Autodesk Inventor part; units mm, degrees
(part 2 of 2)
sketch "Sketch11" plane through (0, 0, 0) normal (0, -1, 0) x (1, 0, 0)
  line L0 (38.5, 57.5) -> (38.5, -57.5) construction
  line L1 (-38.5, 57.5) -> (38.5, 57.5) construction
  line L2 (-38.5, 57.5) -> (-38.5, -57.5) construction
  line L3 (-38.5, -57.5) -> (38.5, -57.5) construction
  line L4 (-32.0325, -46.9289) -> (-28.4969, -50.4645)
  line L5 (-28.4969, -50.4645) -> (-32.0325, -54)
  line L6 (-32.0325, -54) -> (-35.568, -50.4645)
  line L7 (-35.568, -50.4645) -> (-32.0325, -46.9289)
  line L8 (-38.5, -54) -> (-32.0325, -54) construction
  line L9 (31.4645, 54) -> (35, 54) construction
  line L10 (-38.5, -54) -> (35, -54) construction
  line L11 (35, 54) -> (-38.5, 54)
  line L12 (-38.5, 54) -> (-38.5, -54) construction
  line L13 (-22.9615, -46.9289) -> (-19.4259, -50.4645)
  line L14 (-26.497, -50.4645) -> (-22.9615, -46.9289)
  line L15 (-19.4259, -50.4645) -> (-22.9615, -54)
  line L16 (-22.9615, -54) -> (-26.497, -50.4645)
  line L17 (-13.8905, -46.9289) -> (-10.3549, -50.4645)
  line L18 (-17.426, -50.4645) -> (-13.8905, -46.9289)
  line L19 (-10.3549, -50.4645) -> (-13.8905, -54)
  line L20 (-13.8905, -54) -> (-17.426, -50.4645)
  line L21 (-4.8195, -46.9289) -> (-1.2839, -50.4645)
  line L22 (-8.355, -50.4645) -> (-4.8195, -46.9289)
  line L23 (-1.2839, -50.4645) -> (-4.8195, -54)
  line L24 (-4.8195, -54) -> (-8.355, -50.4645)
  line L25 (4.2515, -46.9289) -> (7.7871, -50.4645)
  line L26 (0.716, -50.4645) -> (4.2515, -46.9289)
  line L27 (7.7871, -50.4645) -> (4.2515, -54)
  line L28 (4.2515, -54) -> (0.716, -50.4645)
  line L29 (13.3225, -46.9289) -> (16.8581, -50.4645)
  line L30 (9.787, -50.4645) -> (13.3225, -46.9289)
  line L31 (16.8581, -50.4645) -> (13.3225, -54)
  line L32 (13.3225, -54) -> (9.787, -50.4645)
  line L33 (22.3935, -46.9289) -> (25.9291, -50.4645)
  line L34 (18.858, -50.4645) -> (22.3935, -46.9289)
  line L35 (25.9291, -50.4645) -> (22.3935, -54)
  line L36 (22.3935, -54) -> (18.858, -50.4645)
  line L37 (31.4645, -46.9289) -> (35.0001, -50.4645)
  line L38 (27.929, -50.4645) -> (31.4645, -46.9289)
  line L39 (35.0001, -50.4645) -> (31.4645, -54)
  line L40 (31.4645, -54) -> (27.929, -50.4645)
  line L41 (-32.0325, -37.9489) -> (-28.4969, -41.4845)
  line L42 (-35.568, -41.4845) -> (-32.0325, -37.9489)
  line L43 (-28.4969, -41.4845) -> (-32.0325, -45.02)
  line L44 (-32.0325, -45.02) -> (-35.568, -41.4845)
  line L45 (-22.9615, -37.9489) -> (-19.4259, -41.4845)
  line L46 (-26.497, -41.4845) -> (-22.9615, -37.9489)
  line L47 (-19.4259, -41.4845) -> (-22.9615, -45.02)
  line L48 (-22.9615, -45.02) -> (-26.497, -41.4845)
  line L49 (-13.8905, -37.9489) -> (-10.3549, -41.4845)
  line L50 (-17.426, -41.4845) -> (-13.8905, -37.9489)
  line L51 (-10.3549, -41.4845) -> (-13.8905, -45.02)
  line L52 (-13.8905, -45.02) -> (-17.426, -41.4845)
  line L53 (-4.8195, -37.9489) -> (-1.2839, -41.4845)
  line L54 (-8.355, -41.4845) -> (-4.8195, -37.9489)
  line L55 (-1.2839, -41.4845) -> (-4.8195, -45.02)
  line L56 (-4.8195, -45.02) -> (-8.355, -41.4845)
  line L57 (4.2515, -37.9489) -> (7.7871, -41.4845)
  line L58 (0.716, -41.4845) -> (4.2515, -37.9489)
  line L59 (7.7871, -41.4845) -> (4.2515, -45.02)
  line L60 (4.2515, -45.02) -> (0.716, -41.4845)
  line L61 (13.3225, -37.9489) -> (16.8581, -41.4845)
  line L62 (9.787, -41.4845) -> (13.3225, -37.9489)
  line L63 (16.8581, -41.4845) -> (13.3225, -45.02)
  line L64 (13.3225, -45.02) -> (9.787, -41.4845)
  line L65 (22.3935, -37.9489) -> (25.9291, -41.4845)
  line L66 (18.858, -41.4845) -> (22.3935, -37.9489)
  line L67 (25.9291, -41.4845) -> (22.3935, -45.02)
  line L68 (22.3935, -45.02) -> (18.858, -41.4845)
  line L69 (31.4645, -37.9489) -> (35.0001, -41.4845)
  line L70 (27.929, -41.4845) -> (31.4645, -37.9489)
  line L71 (35.0001, -41.4845) -> (31.4645, -45.02)
  line L72 (31.4645, -45.02) -> (27.929, -41.4845)
  line L73 (-32.0325, -28.9689) -> (-28.4969, -32.5045)
  line L74 (-35.568, -32.5045) -> (-32.0325, -28.9689)
  line L75 (-28.4969, -32.5045) -> (-32.0325, -36.04)
  line L76 (-32.0325, -36.04) -> (-35.568, -32.5045)
  line L77 (-22.9615, -28.9689) -> (-19.4259, -32.5045)
  line L78 (-26.497, -32.5045) -> (-22.9615, -28.9689)
  line L79 (-19.4259, -32.5045) -> (-22.9615, -36.04)
  line L80 (-22.9615, -36.04) -> (-26.497, -32.5045)
  line L81 (-13.8905, -28.9689) -> (-10.3549, -32.5045)
  line L82 (-17.426, -32.5045) -> (-13.8905, -28.9689)
  line L83 (-10.3549, -32.5045) -> (-13.8905, -36.04)
  line L84 (-13.8905, -36.04) -> (-17.426, -32.5045)
  line L85 (-4.8195, -28.9689) -> (-1.2839, -32.5045)
  line L86 (-8.355, -32.5045) -> (-4.8195, -28.9689)
  line L87 (-1.2839, -32.5045) -> (-4.8195, -36.04)
  line L88 (-4.8195, -36.04) -> (-8.355, -32.5045)
  line L89 (4.2515, -28.9689) -> (7.7871, -32.5045)
  line L90 (0.716, -32.5045) -> (4.2515, -28.9689)
  line L91 (7.7871, -32.5045) -> (4.2515, -36.04)
  line L92 (4.2515, -36.04) -> (0.716, -32.5045)
  line L93 (13.3225, -28.9689) -> (16.8581, -32.5045)
  line L94 (9.787, -32.5045) -> (13.3225, -28.9689)
  line L95 (16.8581, -32.5045) -> (13.3225, -36.04)
  line L96 (13.3225, -36.04) -> (9.787, -32.5045)
  line L97 (22.3935, -28.9689) -> (25.9291, -32.5045)
  line L98 (18.858, -32.5045) -> (22.3935, -28.9689)
  line L99 (25.9291, -32.5045) -> (22.3935, -36.04)
  line L100 (22.3935, -36.04) -> (18.858, -32.5045)
  line L101 (31.4645, -28.9689) -> (35.0001, -32.5045)
  line L102 (27.929, -32.5045) -> (31.4645, -28.9689)
  line L103 (35.0001, -32.5045) -> (31.4645, -36.04)
  line L104 (31.4645, -36.04) -> (27.929, -32.5045)
  line L105 (-32.0325, -19.9889) -> (-28.4969, -23.5245)
  line L106 (-35.568, -23.5245) -> (-32.0325, -19.9889)
  line L107 (-28.4969, -23.5245) -> (-32.0325, -27.06)
  line L108 (-32.0325, -27.06) -> (-35.568, -23.5245)
  line L109 (-22.9615, -19.9889) -> (-19.4259, -23.5245)
  line L110 (-26.497, -23.5245) -> (-22.9615, -19.9889)
  line L111 (-19.4259, -23.5245) -> (-22.9615, -27.06)
  line L112 (-22.9615, -27.06) -> (-26.497, -23.5245)
  line L113 (-13.8905, -19.9889) -> (-10.3549, -23.5245)
  line L114 (-17.426, -23.5245) -> (-13.8905, -19.9889)
  line L115 (-10.3549, -23.5245) -> (-13.8905, -27.06)
  line L116 (-13.8905, -27.06) -> (-17.426, -23.5245)
  line L117 (-4.8195, -19.9889) -> (-1.2839, -23.5245)
  line L118 (-8.355, -23.5245) -> (-4.8195, -19.9889)
  line L119 (-1.2839, -23.5245) -> (-4.8195, -27.06)
  line L120 (-4.8195, -27.06) -> (-8.355, -23.5245)
  line L121 (4.2515, -19.9889) -> (7.7871, -23.5245)
  line L122 (0.716, -23.5245) -> (4.2515, -19.9889)
  line L123 (7.7871, -23.5245) -> (4.2515, -27.06)
  line L124 (4.2515, -27.06) -> (0.716, -23.5245)
  line L125 (13.3225, -19.9889) -> (16.8581, -23.5245)
  line L126 (9.787, -23.5245) -> (13.3225, -19.9889)
  line L127 (16.8581, -23.5245) -> (13.3225, -27.06)
  line L128 (13.3225, -27.06) -> (9.787, -23.5245)
  line L129 (22.3935, -19.9889) -> (25.9291, -23.5245)
  line L130 (18.858, -23.5245) -> (22.3935, -19.9889)
  line L131 (25.9291, -23.5245) -> (22.3935, -27.06)
  line L132 (22.3935, -27.06) -> (18.858, -23.5245)
  line L133 (31.4645, -19.9889) -> (35.0001, -23.5245)
  line L134 (27.929, -23.5245) -> (31.4645, -19.9889)
  line L135 (35.0001, -23.5245) -> (31.4645, -27.06)
  line L136 (31.4645, -27.06) -> (27.929, -23.5245)
  line L137 (-32.0325, -11.0089) -> (-28.4969, -14.5445)
  line L138 (-35.568, -14.5445) -> (-32.0325, -11.0089)
  line L139 (-28.4969, -14.5445) -> (-32.0325, -18.08)
  line L140 (-32.0325, -18.08) -> (-35.568, -14.5445)
  line L141 (-22.9615, -11.0089) -> (-19.4259, -14.5445)
  line L142 (-26.497, -14.5445) -> (-22.9615, -11.0089)
  line L143 (-19.4259, -14.5445) -> (-22.9615, -18.08)
  line L144 (-22.9615, -18.08) -> (-26.497, -14.5445)
  line L145 (-13.8905, -11.0089) -> (-10.3549, -14.5445)
  line L146 (-17.426, -14.5445) -> (-13.8905, -11.0089)
  line L147 (-10.3549, -14.5445) -> (-13.8905, -18.08)
  line L148 (-13.8905, -18.08) -> (-17.426, -14.5445)
  line L149 (-4.8195, -11.0089) -> (-1.2839, -14.5445)
  line L150 (-8.355, -14.5445) -> (-4.8195, -11.0089)
  line L151 (-1.2839, -14.5445) -> (-4.8195, -18.08)
  line L152 (-4.8195, -18.08) -> (-8.355, -14.5445)
  line L153 (4.2515, -11.0089) -> (7.7871, -14.5445)
  line L154 (0.716, -14.5445) -> (4.2515, -11.0089)
  line L155 (7.7871, -14.5445) -> (4.2515, -18.08)
  line L156 (4.2515, -18.08) -> (0.716, -14.5445)
  line L157 (13.3225, -11.0089) -> (16.8581, -14.5445)
  line L158 (9.787, -14.5445) -> (13.3225, -11.0089)
  line L159 (16.8581, -14.5445) -> (13.3225, -18.08)
  line L160 (13.3225, -18.08) -> (9.787, -14.5445)
  line L161 (22.3935, -11.0089) -> (25.9291, -14.5445)
  line L162 (18.858, -14.5445) -> (22.3935, -11.0089)
  line L163 (25.9291, -14.5445) -> (22.3935, -18.08)
  line L164 (22.3935, -18.08) -> (18.858, -14.5445)
  line L165 (31.4645, -11.0089) -> (35.0001, -14.5445)
  line L166 (27.929, -14.5445) -> (31.4645, -11.0089)
  line L167 (35.0001, -14.5445) -> (31.4645, -18.08)
  line L168 (31.4645, -18.08) -> (27.929, -14.5445)
  line L169 (-38.5, -57.5) -> (-38.5, 57.5) construction
  line L170 (-38.5, 0) -> (38.5, 0) construction
  line L171 (38.5, 57.5) -> (38.5, -57.5) construction
  line L172 (-31.0325, -45.9745) -> (-27.497, -49.51)
  line L173 (-27.497, -49.51) -> (-23.9614, -45.9745)
  line L174 (-23.9614, -45.9745) -> (-27.497, -42.4389)
  line L175 (-27.497, -42.4389) -> (-31.0325, -45.9745)
  line L176 (-18.426, -49.51) -> (-14.8904, -45.9745)
  line L177 (-14.8904, -45.9745) -> (-18.426, -42.4389)
  line L178 (-21.9615, -45.9745) -> (-18.426, -49.51)
  line L179 (-18.426, -42.4389) -> (-21.9615, -45.9745)
  line L180 (-9.355, -49.51) -> (-5.8194, -45.9745)
  line L181 (-5.8194, -45.9745) -> (-9.355, -42.4389)
  line L182 (-12.8905, -45.9745) -> (-9.355, -49.51)
  line L183 (-9.355, -42.4389) -> (-12.8905, -45.9745)
  line L184 (-0.284, -49.51) -> (3.2516, -45.9745)
  line L185 (3.2516, -45.9745) -> (-0.284, -42.4389)
  line L186 (-3.8195, -45.9745) -> (-0.284, -49.51)
  line L187 (-0.284, -42.4389) -> (-3.8195, -45.9745)
  line L188 (8.787, -49.51) -> (12.3226, -45.9745)
  line L189 (12.3226, -45.9745) -> (8.787, -42.4389)
  line L190 (5.2515, -45.9745) -> (8.787, -49.51)
  line L191 (8.787, -42.4389) -> (5.2515, -45.9745)
  line L192 (17.858, -49.51) -> (21.3936, -45.9745)
  line L193 (21.3936, -45.9745) -> (17.858, -42.4389)
  line L194 (14.3225, -45.9745) -> (17.858, -49.51)
  line L195 (17.858, -42.4389) -> (14.3225, -45.9745)
  line L196 (26.929, -49.51) -> (30.4646, -45.9745)
  line L197 (30.4646, -45.9745) -> (26.929, -42.4389)
  line L198 (23.3935, -45.9745) -> (26.929, -49.51)
  line L199 (26.929, -42.4389) -> (23.3935, -45.9745)
  line L200 (-27.497, -40.53) -> (-23.9614, -36.9945)
  line L201 (-23.9614, -36.9945) -> (-27.497, -33.4589)
  line L202 (-31.0325, -36.9945) -> (-27.497, -40.53)
  line L203 (-27.497, -33.4589) -> (-31.0325, -36.9945)
  line L204 (-18.426, -40.53) -> (-14.8904, -36.9945)
  line L205 (-14.8904, -36.9945) -> (-18.426, -33.4589)
  line L206 (-21.9615, -36.9945) -> (-18.426, -40.53)
  line L207 (-18.426, -33.4589) -> (-21.9615, -36.9945)
  line L208 (-9.355, -40.53) -> (-5.8194, -36.9945)
  line L209 (-5.8194, -36.9945) -> (-9.355, -33.4589)
  line L210 (-12.8905, -36.9945) -> (-9.355, -40.53)
  line L211 (-9.355, -33.4589) -> (-12.8905, -36.9945)
  line L212 (-0.284, -40.53) -> (3.2516, -36.9945)
  line L213 (3.2516, -36.9945) -> (-0.284, -33.4589)
  line L214 (-3.8195, -36.9945) -> (-0.284, -40.53)
  line L215 (-0.284, -33.4589) -> (-3.8195, -36.9945)
  line L216 (8.787, -40.53) -> (12.3226, -36.9945)
  line L217 (12.3226, -36.9945) -> (8.787, -33.4589)
  line L218 (5.2515, -36.9945) -> (8.787, -40.53)
  line L219 (8.787, -33.4589) -> (5.2515, -36.9945)
  line L220 (17.858, -40.53) -> (21.3936, -36.9945)
  line L221 (21.3936, -36.9945) -> (17.858, -33.4589)
  line L222 (14.3225, -36.9945) -> (17.858, -40.53)
  line L223 (17.858, -33.4589) -> (14.3225, -36.9945)
  line L224 (26.929, -40.53) -> (30.4646, -36.9945)
  line L225 (30.4646, -36.9945) -> (26.929, -33.4589)
  line L226 (23.3935, -36.9945) -> (26.929, -40.53)
  line L227 (26.929, -33.4589) -> (23.3935, -36.9945)
  line L228 (-27.497, -31.55) -> (-23.9614, -28.0145)
  line L229 (-23.9614, -28.0145) -> (-27.497, -24.4789)
  line L230 (-31.0325, -28.0145) -> (-27.497, -31.55)
  line L231 (-27.497, -24.4789) -> (-31.0325, -28.0145)
  line L232 (-18.426, -31.55) -> (-14.8904, -28.0145)
  line L233 (-14.8904, -28.0145) -> (-18.426, -24.4789)
  line L234 (-21.9615, -28.0145) -> (-18.426, -31.55)
  line L235 (-18.426, -24.4789) -> (-21.9615, -28.0145)
  line L236 (-9.355, -31.55) -> (-5.8194, -28.0145)
  line L237 (-5.8194, -28.0145) -> (-9.355, -24.4789)
  line L238 (-12.8905, -28.0145) -> (-9.355, -31.55)
  line L239 (-9.355, -24.4789) -> (-12.8905, -28.0145)
  line L240 (-0.284, -31.55) -> (3.2516, -28.0145)
  line L241 (3.2516, -28.0145) -> (-0.284, -24.4789)
  line L242 (-3.8195, -28.0145) -> (-0.284, -31.55)
  line L243 (-0.284, -24.4789) -> (-3.8195, -28.0145)
  line L244 (8.787, -31.55) -> (12.3226, -28.0145)
  line L245 (12.3226, -28.0145) -> (8.787, -24.4789)
  line L246 (5.2515, -28.0145) -> (8.787, -31.55)
  line L247 (8.787, -24.4789) -> (5.2515, -28.0145)
  line L248 (17.858, -31.55) -> (21.3936, -28.0145)
  line L249 (21.3936, -28.0145) -> (17.858, -24.4789)
  line L250 (14.3225, -28.0145) -> (17.858, -31.55)
  line L251 (17.858, -24.4789) -> (14.3225, -28.0145)
  line L252 (26.929, -31.55) -> (30.4646, -28.0145)
  line L253 (30.4646, -28.0145) -> (26.929, -24.4789)
  line L254 (23.3935, -28.0145) -> (26.929, -31.55)
  line L255 (26.929, -24.4789) -> (23.3935, -28.0145)
  line L256 (-27.497, -22.57) -> (-23.9614, -19.0345)
  line L257 (-23.9614, -19.0345) -> (-27.497, -15.4989)
  line L258 (-31.0325, -19.0345) -> (-27.497, -22.57)
  line L259 (-27.497, -15.4989) -> (-31.0325, -19.0345)
  line L260 (-18.426, -22.57) -> (-14.8904, -19.0345)
  line L261 (-14.8904, -19.0345) -> (-18.426, -15.4989)
  line L262 (-21.9615, -19.0345) -> (-18.426, -22.57)
  line L263 (-18.426, -15.4989) -> (-21.9615, -19.0345)
  line L264 (-9.355, -22.57) -> (-5.8194, -19.0345)
  line L265 (-5.8194, -19.0345) -> (-9.355, -15.4989)
  line L266 (-12.8905, -19.0345) -> (-9.355, -22.57)
  line L267 (-9.355, -15.4989) -> (-12.8905, -19.0345)
  line L268 (-0.284, -22.57) -> (3.2516, -19.0345)
  line L269 (3.2516, -19.0345) -> (-0.284, -15.4989)
  line L270 (-3.8195, -19.0345) -> (-0.284, -22.57)
  line L271 (-0.284, -15.4989) -> (-3.8195, -19.0345)
  line L272 (8.787, -22.57) -> (12.3226, -19.0345)
  line L273 (12.3226, -19.0345) -> (8.787, -15.4989)
  line L274 (5.2515, -19.0345) -> (8.787, -22.57)
  line L275 (8.787, -15.4989) -> (5.2515, -19.0345)
  line L276 (17.858, -22.57) -> (21.3936, -19.0345)
  line L277 (21.3936, -19.0345) -> (17.858, -15.4989)
  line L278 (14.3225, -19.0345) -> (17.858, -22.57)
  line L279 (17.858, -15.4989) -> (14.3225, -19.0345)
  line L280 (26.929, -22.57) -> (30.4646, -19.0345)
  line L281 (30.4646, -19.0345) -> (26.929, -15.4989)
  line L282 (23.3935, -19.0345) -> (26.929, -22.57)
  line L283 (26.929, -15.4989) -> (23.3935, -19.0345)
  line L284 (33.41, -11) -> (35, -11)
  line L285 (35, -11) -> (35, -12.59)
  line L286 (24.339, -11) -> (29.519, -11)
  line L287 (35, -12.59) -> (33.41, -11)
  line L288 (24.339, -11) -> (26.929, -13.59)
  line L289 (26.929, -13.59) -> (29.519, -11)
  line L290 (15.268, -11) -> (17.858, -13.59)
  line L291 (17.858, -13.59) -> (20.448, -11)
  line L292 (15.268, -11) -> (20.448, -11)
  line L293 (6.197, -11) -> (8.787, -13.59)
  line L294 (8.787, -13.59) -> (11.377, -11)
  line L295 (6.197, -11) -> (11.377, -11)
  line L296 (-2.874, -11) -> (-0.284, -13.59)
  line L297 (-0.284, -13.59) -> (2.306, -11)
  line L298 (-2.874, -11) -> (2.306, -11)
  line L299 (-11.945, -11) -> (-9.355, -13.59)
  line L300 (-9.355, -13.59) -> (-6.765, -11)
  line L301 (-11.945, -11) -> (-6.765, -11)
  line L302 (-21.016, -11) -> (-18.426, -13.59)
  line L303 (-18.426, -13.59) -> (-15.836, -11)
  line L304 (-21.016, -11) -> (-15.836, -11)
  line L305 (-30.087, -11) -> (-27.497, -13.59)
  line L306 (-27.497, -13.59) -> (-24.907, -11)
  line L307 (-30.087, -11) -> (-24.907, -11)
  line L308 (-45.6598, -32.5) -> (56.4301, -32.5) construction
  line L309 (-35.568, -21.57) -> (-33.0324, -19.0345)
  line L310 (-33.0324, -19.0345) -> (-35.568, -16.4989)
  line L311 (-35.568, -21.57) -> (-35.568, -16.4989)
  line L312 (-35.568, -30.55) -> (-33.0324, -28.0145)
  line L313 (-33.0324, -28.0145) -> (-35.568, -25.4789)
  line L314 (-35.568, -30.55) -> (-35.568, -25.4789)
  line L315 (-35.568, -12.59) -> (-33.978, -11)
  line L316 (-35.568, -12.59) -> (-35.568, -11)
  line L317 (-35.568, -11) -> (-33.978, -11)
  line L318 (-0.284, -80.4638) -> (-0.284, 80.7093) construction
  line L319 (35.0001, -21.57) -> (32.4645, -19.0345)
  line L320 (32.4645, -19.0345) -> (35.0001, -16.4989)
  line L321 (35.0001, -21.57) -> (35.0001, -16.4989)
  line L322 (35.0001, -30.55) -> (32.4645, -28.0145)
  line L323 (32.4645, -28.0145) -> (35.0001, -25.4789)
  line L324 (35.0001, -30.55) -> (35.0001, -25.4789)
  line L325 (-35.568, -43.43) -> (-33.0324, -45.9655)
  line L326 (-33.0324, -45.9655) -> (-35.568, -48.5011)
  line L327 (-35.568, -43.43) -> (-35.568, -48.5011)
  line L328 (-35.568, -34.45) -> (-33.0324, -36.9855)
  line L329 (-33.0324, -36.9855) -> (-35.568, -39.5211)
  line L330 (-35.568, -34.45) -> (-35.568, -39.5211)
  line L331 (-35.568, -52.41) -> (-33.978, -54)
  line L332 (-35.568, -52.41) -> (-35.568, -54)
  line L333 (-35.568, -54) -> (-33.978, -54)
  line L334 (24.339, -54) -> (29.519, -54)
  line L335 (24.339, -54) -> (26.929, -51.41)
  line L336 (26.929, -51.41) -> (29.519, -54)
  line L337 (15.268, -54) -> (17.858, -51.41)
  line L338 (17.858, -51.41) -> (20.448, -54)
  line L339 (15.268, -54) -> (20.448, -54)
  line L340 (6.197, -54) -> (8.787, -51.41)
  line L341 (8.787, -51.41) -> (11.377, -54)
  line L342 (6.197, -54) -> (11.377, -54)
  line L343 (-2.874, -54) -> (-0.284, -51.41)
  line L344 (-0.284, -51.41) -> (2.306, -54)
  line L345 (-2.874, -54) -> (2.306, -54)
  line L346 (-11.945, -54) -> (-9.355, -51.41)
  line L347 (-9.355, -51.41) -> (-6.765, -54)
  line L348 (-11.945, -54) -> (-6.765, -54)
  line L349 (-21.016, -54) -> (-18.426, -51.41)
  line L350 (-18.426, -51.41) -> (-15.836, -54)
  line L351 (-21.016, -54) -> (-15.836, -54)
  line L352 (-30.087, -54) -> (-27.497, -51.41)
  line L353 (-27.497, -51.41) -> (-24.907, -54)
  line L354 (-30.087, -54) -> (-24.907, -54)
  line L355 (33.41, -54) -> (35, -54)
  line L356 (35, -54) -> (35, -52.41)
  line L357 (35, -52.41) -> (33.41, -54)
  line L358 (35.0001, -34.45) -> (32.4645, -36.9855)
  line L359 (32.4645, -36.9855) -> (35.0001, -39.5211)
  line L360 (35.0001, -34.45) -> (35.0001, -39.5211)
  line L361 (35.0001, -43.43) -> (35.0001, -48.5011)
  line L362 (32.4645, -45.9655) -> (35.0001, -48.5011)
  line L363 (35.0001, -43.43) -> (32.4645, -45.9655)
  point P0 (0, 0)
  dimension "d88" = 5
  dimension "d89" = 5
  dimension "d91" = 3.5
  dimension "d93" = 3.5
  dimension "d94" = 2.932
  dimension "d95" = 108
  dimension "d96" = 7.0711
  dimension "d100" = 9.071
  dimension "d103" = 8.98
  dimension "d106" = 5
  dimension "d107" = 5
  dimension "d108" = 1.382
  dimension "d109" = 1.382
  dimension "d110" = 1.382
  dimension "d111" = 1.382
  dimension "d114" = 9.071
  dimension "d117" = 8.98
  dimension "d120" = 1.382
  dimension "d121" = 1.382
  dimension "d122" = 1.382
  dimension "d123" = 90
  dimension "d126" = 9.071
  dimension "d132" = 21.5
  dimension "d134" = 1.382
  dimension "d135" = 1.382
  dimension "d136" = 1.382
  dimension "d140" = 1.382
  dimension "d141" = 1.382
  dimension "d144" = 1.382
  dimension "d145" = 0
  constraints: 712 end point, 52 symmetric about line, 14 point on line, 6 parallel, 6 vertical, 5 horizontal, 3 perpendicular, 2 midpoint, 570 other
  measures "d88" distance between parallel lines of L6 L4
  measures "d89" distance between parallel lines of L7 L5
  measures "d91" distance from line of L3 L5.end
  measures "d93" distance between parallel lines of L1 L11
  measures "d94" distance from line of L2 L6.end
  measures "d95" distance between parallel lines of L11 L8
  measures "d96" distance of L4.start L8.end
  measures "d100" distance of L4.start L13.start
  measures "d103" distance of L4.start L41.start
  measures "d106" distance between parallel lines of L175 L173
  measures "d107" distance between parallel lines of L172 L174
  measures "d108" distance between parallel lines of L4 L172
  measures "d109" distance between parallel lines of L48 L174
  measures "d110" distance between parallel lines of L43 L175
  measures "d111" distance between parallel lines of L14 L173
  measures "d114" distance of L172.end L176.start
  measures "d117" distance of L172.end L200.start
  measures "d120" distance between parallel lines of L287 L165
  measures "d121" distance between parallel lines of L288 L161
  measures "d122" distance between parallel lines of L166 L289
  measures "d123" angle of L289 L288
  measures "d126" distance of L288.start L290.start
  measures "d132" distance between parallel lines of L8 L308
  measures "d134" distance between parallel lines of L309 L106
  measures "d135" distance between parallel lines of L258 L105
  measures "d136" distance between parallel lines of L140 L310
  measures "d140" distance between parallel lines of L312 L74
  measures "d141" distance between parallel lines of L108 L313
  measures "d144" distance between parallel lines of L315 L138
  measures "d145" distance from line of L318 L268.start
body "Solid1"
